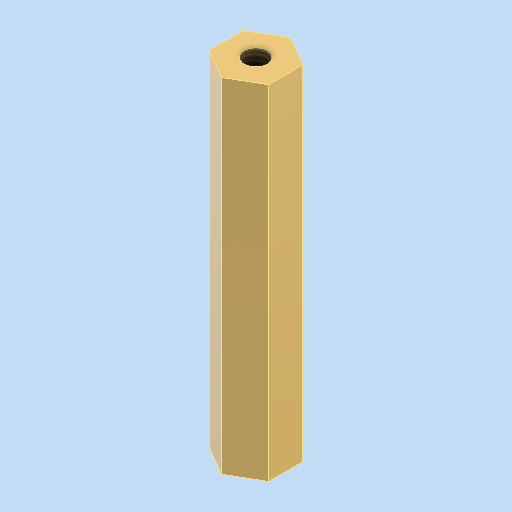
# Autodesk Inventor part: втулки крепления электроники
Saved by Autodesk Inventor 2025 (Build 290162000, 162)
## iProperties
Created: 2025-03-03
Part Number: втулки крепления электроники
Material: Бронза
Document SubType Name: Modeling
Designer: volko
Density: 8.47 g/cm^3
Appearance: Бронза — полированная
Author: volko
Autodesk Inventor part; units mm, degrees
ref_plane "YZ Plane" through (0, 0, 0) normal (1, 0, 0) x (0, 1, 0)
ref_plane "XZ Plane" through (0, 0, 0) normal (0, 1, 0) x (-1, 0, 0)
ref_plane "XY Plane" through (0, 0, 0) normal (0, 0, 1) x (1, 0, 0)
sketch "Эскиз1" plane through (0, 0, 0) normal (0, 1, 0) x (-1, 0, 0)
  line L0 (0, -3) -> (-2.5981, -1.5)
  line L1 (-2.5981, -1.5) -> (-2.5981, 1.5)
  line L2 (-2.5981, 1.5) -> (0, 3)
  line L3 (0, 3) -> (2.5981, 1.5)
  line L4 (2.5981, 1.5) -> (2.5981, -1.5)
  line L5 (2.5981, -1.5) -> (0, -3)
  circle A0 centre (0, 0) radius 3 construction
  dimension "d0" = 6
  constraints: 12 end point, 2 coincident, 1 vertical, 1 vertical alignment, 15 other
extrude "Выдавливание1" add sketch "Эскиз1" along normal blind 30
sketch "Эскиз2" plane through (0, 30, 0) normal (0, 1, 0) x (1, 0, 0)
  point P0 (0, 0)
  point P1 (-0.0431, 0.0216)
hole "Отверстие1" at (-0.0431, 30, -0.0216) direction (0, -1, 0) diameter 2.013 end through all thread size "M2.5x0.45" class "6H" standard "ISO Metric profile"
